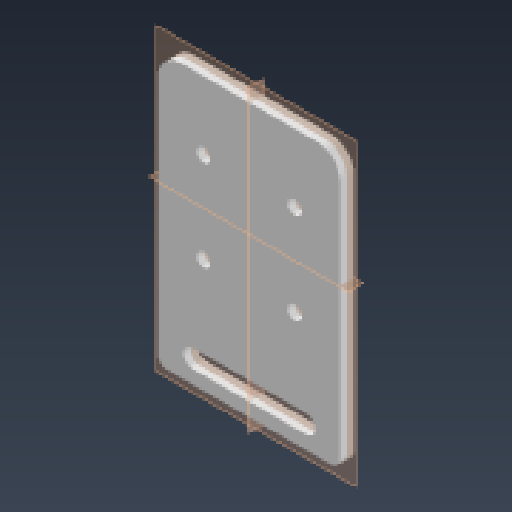
# Autodesk Inventor part: Фанерка_маркера
Saved by Autodesk Inventor 2023.2 (Build 272271030, 271C)
## iProperties
Created: 2026-01-04
Part Number: Фанерка_маркера
Material: Типовые
Document SubType Name: Modeling
Designer: Олег Коноваленко
Density: 1 g/cm^3
Appearance: По умолчанию
Author: Олег Коноваленко
Autodesk Inventor part; units mm, degrees
sketch "Эскиз1" plane through (0, 0, 0) normal (0, 0, 1) x (1, 0, 0)
  line L0 (-20, 25) -> (20, 25)
  line L1 (20, 25) -> (20, -25)
  line L2 (20, -25) -> (-20, -25)
  line L3 (-20, -25) -> (-20, 25)
  line L4 (-20, 25) -> (20, -25) construction
  line L5 (20, 25) -> (-20, -25) construction
  point P0 (0, 0)
  dimension "d1" = 40
  dimension "d10" = 50
  constraints: 12 end point, 2 midpoint, 2 parallel, 1 horizontal, 1 perpendicular
  measures "d1" distance of L1.end L2.end
  measures "d10" distance of L0.end L1.end
extrude "Выдавливание1" add sketch "Эскиз1" along normal mid plane 3
fillet "Сопряжение1" radius 5 2 edges at (20, 25, 0) (-20, 25, 0)
sketch "Эскиз4" plane through (-20, -25, 1.5) normal (0, -1, 0) x (1, 0, 0)
  line L0 (40, -3) -> (40, 0) projected
  line L1 (0, 0) -> (40, 0) projected
  line L2 (0, 0) -> (0, -3) projected
  line L3 (40, -3) -> (0, -3) projected
  point P0 (20, -1.5)
extrude "Выдавливание4" add sketch "Эскиз4" along normal blind 10
sketch "Эскиз5" plane through (0, 0, -1.5) normal (0, 0, -1) x (-1, 0, 0)
  line L0 (12.5, -30) -> (-12.5, -30) construction
  line L1 (12.5, -28) -> (-12.5, -28)
  line L2 (-12.5, -32) -> (12.5, -32)
  arc A0 (12.5, -32) -> (12.5, -28) centre (12.5, -30) ccw
  arc A1 (-12.5, -28) -> (-12.5, -32) centre (-12.5, -30) ccw
  line L3 (0, -47) -> (0, 37) construction
  line L4 (20, -35) -> (-20, -35) projected
  point P0 (0, 0)
  point P1 (0, -30)
  dimension "d20" = 2
  dimension "d21" = 25
  dimension "d22" = 3
  constraints: 8 end point, 4 point on circle, 4 tangent, 2 centre point, 1 horizontal, 1 midpoint, 1 parallel, 1 point on line
  measures "d20" distance between parallel lines of L0 L2
  measures "d21" distance of L0.start L0.end
  measures "d22" distance between parallel lines of L4 L2
extrude "Выдавливание5" cut sketch "Эскиз5" against normal up to next
fillet "Сопряжение4" radius 2 2 edges at (-20, -35, 0) (20, -35, 0)
sketch "Эскиз6" plane through (0, 0, 1.5) normal (0, 0, 1) x (1, 0, 0)
  circle A0 centre (10, -10) radius 1.5 projected
  circle A1 centre (10, 10) radius 1.5 projected
  circle A2 centre (-10, 10) radius 1.5 projected
  circle A3 centre (-10, -10) radius 1.5 projected
  point P0 (0, 0)
extrude "Выдавливание6" cut sketch "Эскиз6" against normal up to next
